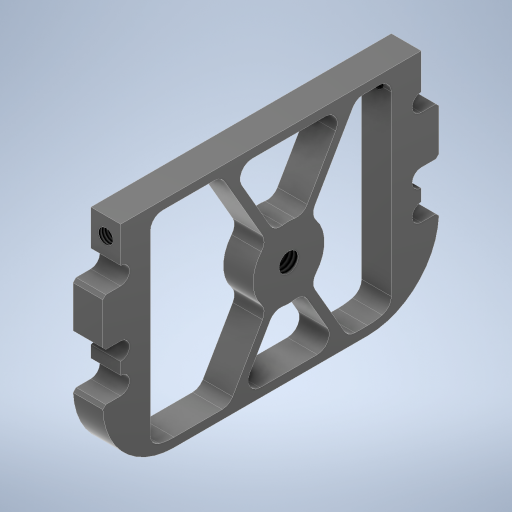
# Autodesk Inventor part: UpperArmIdlerSideFrame
Saved by Autodesk Inventor 2024.2 (Build 282272000, 272)
## iProperties
Created: 2024-01-18
Part Number: UpperArmIdlerSideFrame
Material: Acetal Resin, Black
Document SubType Name: Modeling
Designer: Masato Kubotera
Density: 1.425 g/cm^3
Appearance: Smooth - Black
Mass: 5.1621 g
Surface Area: 38.8553 cm^2
Volume: 3.62252 cm^3
Vendor: meviy
Author: Masato Kubotera
Autodesk Inventor part; units mm, degrees
ref_plane "YZ Plane" through (0, 0, 0) normal (1, 0, 0) x (0, 1, 0)
ref_plane "XZ Plane" through (0, 0, 0) normal (0, 1, 0) x (-1, 0, 0)
derived "UpperArmSideFrameBasis.ipt"
sketch "Sketch1" plane through (0, 0, 0) normal (0, 1, 0) x (-1, 0, 0)
  line L0 (-26, 13.6795) -> (6, 13.6795) construction
  line L1 (6, 13.6795) -> (6, -29.3205) construction
  line L2 (6, -29.3205) -> (-26, -29.3205) construction
  line L3 (-26, -29.3205) -> (-26, 13.6795) construction
  line L4 (-26, 13.6795) -> (6, -29.3205) construction
  line L5 (6, 13.6795) -> (-26, -29.3205) construction
  line L6 (-23.5, 10.6795) -> (3.5, 10.6795) construction
  line L7 (3.5, 10.6795) -> (3.5, -16.3205) construction
  line L8 (3.5, -16.3205) -> (-23.5, -16.3205) construction
  line L9 (-23.5, -16.3205) -> (-23.5, 10.6795) construction
  line L10 (-23.5, 10.6795) -> (3.5, -16.3205) construction
  line L11 (3.5, 10.6795) -> (-23.5, -16.3205) construction
  line L12 (-10, 13.6795) -> (-10, -29.3205) construction
  arc A0 (0.583, -29.3205) -> (6, -17.3205) centre (-10, -17.3205) ccw construction
  circle A1 centre (-10, -17.3205) radius 8 construction
  arc A2 (-26, -17.3205) -> (-20.583, -29.3205) centre (-10, -17.3205) ccw construction
  line L13 (0, 0) -> (-10, -17.3205) construction
  line L14 (-24.4, 13.6795) -> (-24.4, 25.1795) construction
  line L15 (-24.4, 25.1795) -> (4.4, 25.1795) construction
  line L16 (4.4, 25.1795) -> (4.4, 13.6795) construction
  line L17 (-28.25, -17.3205) -> (22.25, -17.3205)
  line L18 (-28.25, -17.3205) -> (-28.25, 19.6795)
  line L19 (-28.25, 19.6795) -> (-19.25, 19.6795)
  line L20 (-28.25, 10.6795) -> (-31.25, 10.6795)
  line L21 (-31.25, 10.6795) -> (-31.25, 2.6795)
  line L22 (-31.25, 2.6795) -> (-28.25, 2.6795)
  arc A3 (-28.25, 10.6795) -> (-28.25, 13.6795) centre (-28.25, 12.1795) ccw
  line L23 (-19.25, 19.6795) -> (19.25, 19.6795)
  line L24 (19.25, 19.6795) -> (22.25, 19.6795)
  line L25 (0, 19.6795) -> (0, -17.3205) construction
  arc A4 (-28.25, -0.3205) -> (-28.25, 2.6795) centre (-28.25, 1.1795) ccw
  line L26 (-3, -17.3205) -> (-3, 19.6795) construction
  line L27 (22.25, 16.6795) -> (16.25, 16.6795) construction
  line L28 (-28.25, 16.6795) -> (-23.25, 16.6795) construction
  line L29 (-26.05, -17.3205) -> (-26.05, 13.6795)
  line L30 (-26.05, 13.6795) -> (6.05, 13.6795)
  line L31 (6.05, 13.6795) -> (6.05, -17.3205)
  arc A5 (-1.5, -17.3205) -> (-18.5, -17.3205) centre (-10, -17.3205) ccw construction
  line L32 (-23.25, 18.1795) -> (-23.25, -15.0288)
  line L33 (9.6299, 18.1795) -> (2.327, 5.5304)
  line L34 (2.327, -5.5304) -> (8.2679, -15.8205)
  line L35 (11.362, 18.1795) -> (3.626, 4.7804)
  line L36 (-3.626, 4.7804) -> (-11.362, 18.1795)
  line L37 (-9.6299, 18.1795) -> (-2.327, 5.5304)
  line L38 (-2.327, -5.5304) -> (-8.2679, -15.8205)
  line L39 (3.626, -4.7804) -> (10, -15.8205)
  arc A6 (-5.6636, -8.3096) -> (-19.8839, -15.8014) centre (-10, -17.3205) ccw
  line L40 (-3.626, -4.7804) -> (-10, -15.8205)
  line L41 (17.25, 18.1795) -> (17.25, -15.0288)
  arc A7 (-0.1131, -15.8205) -> (-4.3646, -9.0596) centre (-10, -17.3205) ccw
  circle A8 centre (3.5, 10.6795) radius 1.55 construction
  line L42 (-23.25, 18.1795) -> (-11.362, 18.1795)
  line L43 (-9.6299, 18.1795) -> (9.6299, 18.1795)
  line L44 (11.362, 18.1795) -> (17.25, 18.1795)
  line L45 (-19.25, -15.8205) -> (-10, -15.8205)
  line L46 (-8.2679, -15.8205) -> (8.2679, -15.8205)
  line L47 (10, -15.8205) -> (13.25, -15.8205)
  arc A9 (-3.626, 4.7804) -> (-3.626, -4.7804) centre (0, 0) ccw
  arc A10 (-2.327, -5.5304) -> (2.327, -5.5304) centre (0, 0) ccw
  arc A11 (3.626, -4.7804) -> (3.626, 4.7804) centre (0, 0) ccw
  arc A12 (2.327, 5.5304) -> (-2.327, 5.5304) centre (0, 0) ccw
  line L48 (-5.2998, 7.6795) -> (-26.0706, 7.6795)
  line L49 (-28.25, -0.3205) -> (-28.25, -2.3205)
  line L50 (-28.25, 19.6795) -> (-28.25, 13.6795)
  line L51 (-31.25, 6.6795) -> (-28.25, 6.6795) construction
  arc A13 (-23.25, -15.0288) -> (-19.25, -15.8205) centre (-19.25, -5.3205) ccw
  line L52 (-19.25, -17.3205) -> (13.25, -17.3205)
  arc A14 (22.25, 13.6795) -> (22.25, 10.6795) centre (22.25, 12.1795) ccw
  line L53 (22.25, 19.6795) -> (22.25, 13.6795)
  line L54 (22.25, 10.6795) -> (25.25, 10.6795)
  line L55 (25.25, 10.6795) -> (25.25, 2.6795)
  line L56 (25.25, 2.6795) -> (22.25, 2.6795)
  line L57 (25.25, 6.6795) -> (22.25, 6.6795) construction
  arc A15 (22.25, 2.6795) -> (22.25, -0.3205) centre (22.25, 1.1795) ccw
  line L58 (22.25, -0.3205) -> (22.25, -2.3205)
  arc A16 (13.25, -15.8205) -> (17.25, -15.0288) centre (13.25, -5.3205) ccw
  line L59 (22.25, 16.6795) -> (17.25, 16.6795) construction
  arc A17 (-28.25, -5.3205) -> (-28.25, -2.3205) centre (-28.25, -3.8205) ccw
  line L60 (-28.25, -5.3205) -> (-31.25, -5.3205)
  arc A18 (-31.25, -5.3205) -> (-19.25, -17.3205) centre (-19.25, -5.3205) ccw
  line L61 (22.25, -5.3205) -> (25.25, -5.3205)
  arc A19 (22.25, -2.3205) -> (22.25, -5.3205) centre (22.25, -3.8205) ccw
  arc A20 (13.25, -17.3205) -> (25.25, -5.3205) centre (13.25, -5.3205) ccw
  line L62 (22.25, -0.3205) -> (22.25, -2.3205)
  point P0 (-10, -7.8205)
  point P1 (-10, -2.8205)
  point P2 (-10, -7.8205)
  point P3 (-28.25, -0.3205)
  point P4 (-1.5, -17.3205)
  point P5 (-1.5, -17.3205)
  point P6 (-6.05, -11.9789)
  point P7 (6.05, 11.9789)
  point P8 (-7.0318, 13.6795)
  point P9 (6.05, -8.9789)
  point P10 (6.05, 8.9789)
  point P11 (6.05, -11.9789)
  point P12 (6.05, -15.8205)
  point P13 (-8.7639, 13.6795)
  point P14 (-23.25, 13.6795)
  point P15 (-29.75, 2.6795)
  point P16 (-28.25, -5.3205)
  point P17 (9.8537, -15.5671)
  point P18 (-28.25, -2.3205)
  point P19 (-28.25, -5.3205)
  point P20 (-19.25, -17.3205)
  point P21 (-28.25, -13.2578)
extrude "Extrusion1" add sketch "Sketch1" along normal blind 5 contours A18 L60 L18 | L18 A17 A4 A3 L19 L23 L24 L53 A14 L54 L55 L56 A15 L58 A19 L61 A20 L17 L31 L46 L34 L39 L47 A16 L41 L44 L35 L33 L43 L37 L30 L36 L42 L32 L29 A18 | A18 L29 L48 L32 A13 L45 L40 A9 L36 L30 L37 A12 L33 L31 L35 A11 L39 L34 A10 L38 L46 L17 | L29 L30 L32 L48 | L22 L21 L20 L18
fillet "Fillet1" radius 2 20 edges at (11.362, 2.5, 18.1795) (23.25, 2.5, 18.1795) (23.25, 2.5, -15.0288) (10, 2.5, -15.8205) (3.626, 2.5, -4.7804) (3.626, 2.5, 4.7804) (-2.327, 2.5, 5.5304) (2.327, 2.5, 5.5304) (9.6299, 2.5, 18.1795) (-9.6299, 2.5, 18.1795) (-11.362, 2.5, 18.1795) (-17.25, 2.5, 18.1795) (-17.25, 2.5, -15.0288) (-10, 2.5, -15.8205) (-8.2679, 2.5, -15.8205) (8.2679, 2.5, -15.8205) (2.327, 2.5, -5.5304) (-2.327, 2.5, -5.5304) (-3.626, 2.5, 4.7804) (-3.626, 2.5, -4.7804)
sketch "Sketch2" plane through (28.25, 0, -0.3205) normal (1, 0, 0) x (0, 0, -1)
  line L0 (-17, 0) -> (-17, 5)
  line L1 (-3, 5) -> (-14, 5) projected
  point P0 (-17, 0)
  point P1 (-20, 5)
  point P2 (-17, 2.5)
  constraints: 2 end point, 1 midpoint, 1 point on line, 1 vertical
chamfer "Chamfer1" distance 0.5 angle 45 6 edges at (31.25, 2.5, 10.6795) (31.25, 2.5, 2.6795) (-25.25, 2.5, 10.6795) (-25.25, 2.5, 2.6795) (31.25, 2.5, -5.3205) (-25.25, 2.5, -5.3205)
hole "M4" at (0, 0, 0) direction (0, 1, 0) diameter 3.242 end through all thread size "M4x0.7" class "6H" standard "ANSI Metric M Profile"
hole "Side-M3" at (28.25, 2.5, 16.6795) direction (-1, 0, 0) diameter 2.459 depth 6 thread size "M3x0.5" class "6H" standard "ANSI Metric M Profile"
ref_plane "Work Plane1" through (3, 0, 13.6795) normal (-1, 0, 0) x (0, 0, 1)
mirror "Mirror1" about plane through (3, 0, 13.6795) normal (-1, 0, 0) of "Side-M3"
body "Solid1"
